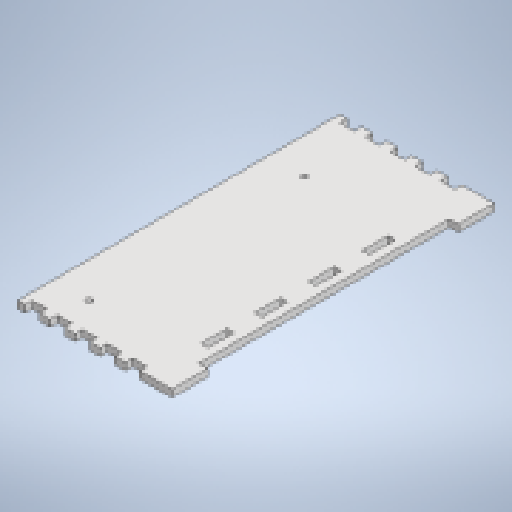
# Autodesk Inventor part: side
Saved by Autodesk Inventor 2025.3 (Build 293356000, 356)
## iProperties
Created: 2025-12-08
Part Number: side
Material: Generic
Document SubType Name: Modeling
Designer: hazem
Density: 1 g/cm^3
Appearance: Default
Author: hazem
Autodesk Inventor part; units mm, degrees
ref_plane "YZ Plane" through (0, 0, 0) normal (1, 0, 0) x (0, 1, 0)
ref_plane "XZ Plane" through (0, 0, 0) normal (0, 1, 0) x (-1, 0, 0)
ref_plane "XY Plane" through (0, 0, 0) normal (0, 0, 1) x (1, 0, 0)
sketch "Sketch1" plane through (0, 0, 0) normal (0, 1, 0) x (-1, 0, 0)
  line L0 (-9.6671, 163.8128) -> (70.4329, 163.8128)
  line L1 (70.4329, 163.8128) -> (70.4329, -16.1872)
  line L2 (70.4329, -16.1872) -> (-9.6671, -16.1872)
  line L3 (-9.6671, -16.1872) -> (-9.6671, 163.8128)
  point P0 (0, 0)
  constraints: 8 end point, 2 parallel, 1 horizontal, 1 perpendicular
extrude "Extrusion1" add sketch "Sketch1" along normal blind 4
sketch "Sketch2" plane through (0, 4, 0) normal (0, 1, 0) x (1, 0, 0)
  line L0 (-66.4329, -159.8128) -> (-66.4329, -148.8128)
  line L1 (-70.4329, -159.8128) -> (-70.4329, -148.8128)
  line L2 (-66.4329, -159.8128) -> (-66.4329, -148.8128) projected
  line L3 (-70.4329, -159.8128) -> (-70.4329, -148.8128) projected
  line L4 (-70.4329, -159.8128) -> (-70.4329, -148.8128) projected
  line L5 (-70.4329, -163.8128) -> (9.6671, -163.8128) projected
  line L6 (-30.3829, -163.8128) -> (-30.3829, 16.1872) construction
  line L7 (9.6671, 16.1872) -> (-70.4329, 16.1872) projected
  line L8 (-70.4329, 0.9372) -> (-66.4329, 0.9372)
  line L9 (-66.4329, -13.5628) -> (-70.4329, -13.5628)
  line L10 (-66.4329, -43.5628) -> (-70.4329, -43.5628)
  line L11 (-70.4329, -29.0628) -> (-66.4329, -29.0628)
  line L12 (-66.4329, -73.5628) -> (-70.4329, -73.5628)
  line L13 (-70.4329, -59.0628) -> (-66.4329, -59.0628)
  line L14 (-66.4329, -103.5628) -> (-70.4329, -103.5628)
  line L15 (-70.4329, -89.0628) -> (-66.4329, -89.0628)
  line L16 (-66.4329, -133.5628) -> (-70.4329, -133.5628)
  line L17 (-70.4329, -119.0628) -> (-66.4329, -119.0628)
  line L18 (5.6671, -159.8128) -> (5.6671, -148.8128)
  line L19 (9.6671, -159.8128) -> (9.6671, -148.8128)
  line L20 (5.6671, -133.8128) -> (5.6671, -118.8128)
  line L21 (9.6671, -133.8128) -> (9.6671, -118.8128)
  line L22 (5.6671, -103.8128) -> (5.6671, -88.8128)
  line L23 (9.6671, -103.8128) -> (9.6671, -88.8128)
  line L24 (5.6671, -73.8128) -> (5.6671, -58.8128)
  line L25 (9.6671, -73.8128) -> (9.6671, -58.8128)
  line L26 (5.6671, -43.8128) -> (5.6671, -28.8128)
  line L27 (9.6671, -43.8128) -> (9.6671, -28.8128)
  line L28 (5.6671, -13.8128) -> (5.6671, 1.1872)
  line L29 (9.6671, -13.8128) -> (9.6671, 1.1872)
  line L30 (9.6671, -149.0628) -> (5.6671, -149.0628)
  line L31 (5.6671, -159.5628) -> (9.6671, -159.5628)
  line L32 (9.6671, 0.9372) -> (5.6671, 0.9372)
  line L33 (5.6671, -13.5628) -> (9.6671, -13.5628)
  line L34 (5.6671, -43.5628) -> (9.6671, -43.5628)
  line L35 (9.6671, -29.0628) -> (5.6671, -29.0628)
  line L36 (5.6671, -73.5628) -> (9.6671, -73.5628)
  line L37 (9.6671, -59.0628) -> (5.6671, -59.0628)
  line L38 (5.6671, -103.5628) -> (9.6671, -103.5628)
  line L39 (9.6671, -89.0628) -> (5.6671, -89.0628)
  line L40 (5.6671, -133.5628) -> (9.6671, -133.5628)
  line L41 (9.6671, -119.0628) -> (5.6671, -119.0628)
  line L42 (-66.4329, -148.8128) -> (-70.4329, -148.8128)
  line L43 (-66.4329, -159.8128) -> (-70.4329, -159.8128)
  line L44 (-66.4329, -148.8128) -> (-70.4329, -148.8128)
  line L45 (-66.4329, -159.8128) -> (-70.4329, -159.8128) projected
  line L46 (-66.4329, -163.8128) -> (-66.4329, -89.0628)
  line L47 (-66.4329, -103.5628) -> (-66.4329, -73.5628)
  line L48 (-66.4329, -89.0628) -> (-66.4329, -43.5628)
  line L49 (-66.4329, -43.5628) -> (-66.4329, -13.5628)
  line L50 (-66.4329, -13.5628) -> (-66.4329, 16.1872)
  line L51 (-70.4329, 16.1872) -> (-70.4329, -163.8128) projected
  line L52 (9.6671, -163.8128) -> (9.6671, 16.1872) projected
  line L53 (1.6671, 16.1872) -> (1.6671, 12.1872)
  line L54 (1.6671, 12.1872) -> (-6.3329, 12.1872)
  line L55 (-6.3329, 12.1872) -> (-6.3329, 16.1872)
  line L56 (-12.3329, 16.1872) -> (-12.3329, 12.1872)
  line L57 (-12.3329, 12.1872) -> (-20.3329, 12.1872)
  line L58 (-20.3329, 12.1872) -> (-20.3329, 16.1872)
  line L59 (-26.3329, 16.1872) -> (-26.3329, 12.1872)
  line L60 (-26.3329, 12.1872) -> (-34.3329, 12.1872)
  line L61 (-34.3329, 12.1872) -> (-34.3329, 16.1872)
  line L62 (-40.3329, 16.1872) -> (-40.3329, 12.1872)
  line L63 (-40.3329, 12.1872) -> (-48.3329, 12.1872)
  line L64 (-48.3329, 12.1872) -> (-48.3329, 16.1872)
  line L65 (-54.3329, 16.1872) -> (-54.3329, 12.1872)
  line L66 (-54.3329, 12.1872) -> (-62.3329, 12.1872)
  line L67 (-62.3329, 12.1872) -> (-62.3329, 16.1872)
  line L68 (-12.3329, -73.8128) -> (-48.4329, -73.8128) construction
  line L69 (1.6671, -163.8128) -> (1.6671, -159.8128)
  line L70 (1.6671, -159.8128) -> (-6.3329, -159.8128)
  line L71 (-6.3329, -159.8128) -> (-6.3329, -163.8128)
  line L72 (-12.3329, -163.8128) -> (-12.3329, -159.8128)
  line L73 (-12.3329, -159.8128) -> (-20.3329, -159.8128)
  line L74 (-20.3329, -159.8128) -> (-20.3329, -163.8128)
  line L75 (-26.3329, -163.8128) -> (-26.3329, -159.8128)
  line L76 (-26.3329, -159.8128) -> (-34.3329, -159.8128)
  line L77 (-34.3329, -159.8128) -> (-34.3329, -163.8128)
  line L78 (-40.3329, -163.8128) -> (-40.3329, -159.8128)
  line L79 (-40.3329, -159.8128) -> (-48.3329, -159.8128)
  line L80 (-48.3329, -159.8128) -> (-48.3329, -163.8128)
  line L81 (-54.3329, -163.8128) -> (-54.3329, -159.8128)
  line L82 (-54.3329, -159.8128) -> (-62.3329, -159.8128)
  line L83 (-62.3329, -159.8128) -> (-62.3329, -163.8128)
  circle A0 centre (-46.4329, -23.8128) radius 1.75
  circle A1 centre (-46.4329, -143.8128) radius 1.75
  point P0 (0, 0)
  point P1 (-66.4329, -43.5628)
  point P2 (-30.3829, -73.8128)
  dimension "d6" = 30
  dimension "d13" = 4
  dimension "d14" = 8
  dimension "d15" = 4
  dimension "d16" = 8
  dimension "d19" = 14
  dimension "d24" = 180
  dimension "d30" = 3.5
  dimension "d32" = 40
  dimension "d34" = 20
  constraints: 152 end point, 44 symmetric about line, 21 point on line, 4 collinear, 4 midpoint, 3 vertical, 2 centre point, 2 horizontal, 1 equal radius, 1 parallel, 1 perpendicular, 1 vertical alignment, 54 other
  measures "d6" distance of L10.start L9.start
  measures "d13" distance of L53.start L53.end
  measures "d14" distance of L53.end L54.end
  measures "d15" distance of L54.end L55.end
  measures "d19" distance of L53.start L56.start
  measures "d24" distance between parallel lines of L5 L7
  measures "d30" diameter of A0
  measures "d32" distance from line of A0.centre L7
  measures "d34" distance from line of L5 A1.centre
extrude "Extrusion2" cut sketch "Sketch2" against normal up to surface (4 mm away) contours L43 L1 L42 L0 | L46 L5 L51 L43 | L42 L51 L16 L46 | L16 L51 L17 L46 | L83 L82 L81 L5 | L17 L51 L14 L46 | L14 L51 L15 L46 | L80 L79 L78 L5 | L15 L51 L12 L47 | L12 L51 L13 L48 | L77 L76 L75 L5 | L13 L51 L10 L48 | L10 L51 L11 L49 | L74 L73 L72 L5 | L11 L51 L9 L49 | L9 L51 L8 L50 | L71 L70 L69 L5 | L8 L51 L7 L50 | L7 L65 L66 L67 | L31 L18 L30 L19 | L7 L62 L63 L64 | L7 L59 L60 L61 | L40 L20 L41 L21 | L7 L56 L57 L58 | L7 L53 L54 L55 | L38 L22 L39 L23 | L29 L33 L28 L32 | L36 L24 L37 L25 | L27 L34 L26 L35 | A0 | A1
sketch "Sketch4" plane through (0, 4, 0) normal (0, 1, 0) x (1, 0, 0)
  line L0 (9.6671, -159.5628) -> (5.6671, -159.5628) projected
  line L1 (9.6671, -149.0628) -> (9.6671, -133.5628) projected
  line L2 (5.6671, -159.5628) -> (9.6671, -159.5628)
  line L3 (9.6671, -159.5628) -> (9.6671, -149.0628)
  line L4 (9.6671, -149.0628) -> (5.6671, -149.0628)
  line L5 (5.6671, -149.0628) -> (5.6671, -159.5628)
  line L6 (5.6671, -13.5628) -> (5.6671, 0.9372) projected
  line L7 (9.6671, -13.5628) -> (5.6671, -13.5628)
  line L8 (5.6671, -13.5628) -> (5.6671, 0.9372)
  line L9 (5.6671, 0.9372) -> (9.6671, 0.9372)
  line L10 (9.6671, 0.9372) -> (9.6671, -133.5628)
  line L11 (9.6671, -13.5628) -> (5.6671, -13.5628) projected
  line L12 (1.6671, -163.8128) -> (9.6671, -163.8128) projected
  line L13 (9.6671, -163.8128) -> (19.6671, -163.8128)
  line L14 (19.6671, -163.8128) -> (19.6671, -143.8128)
  line L15 (19.6671, -143.8128) -> (9.6671, -143.8128)
  line L16 (9.6671, -143.8128) -> (9.6671, -163.8128)
  line L17 (9.6671, 16.1872) -> (1.6671, 16.1872) projected
  line L18 (9.6671, 16.1872) -> (19.6671, 16.1872)
  line L19 (19.6671, 16.1872) -> (19.6671, -3.8128)
  line L20 (19.6671, -3.8128) -> (9.6671, -3.8128)
  line L21 (9.6671, -3.8128) -> (9.6671, 16.1872)
  line L22 (14.6671, -143.8128) -> (14.6671, -3.8128)
  line L23 (-40.3329, -159.8128) -> (-40.3329, -163.8128) projected
  line L24 (-40.3329, -163.8128) -> (-34.3329, -163.8128) projected
  line L25 (-34.3329, -163.8128) -> (-34.3329, -159.8128) projected
  line L26 (-34.3329, -159.8128) -> (-26.3329, -159.8128) projected
  line L27 (-26.3329, -159.8128) -> (-26.3329, -163.8128) projected
  line L28 (-26.3329, -163.8128) -> (-20.3329, -163.8128) projected
  line L29 (-20.3329, -163.8128) -> (-20.3329, -159.8128) projected
  line L30 (-20.3329, -159.8128) -> (-12.3329, -159.8128) projected
  line L31 (-12.3329, -159.8128) -> (-12.3329, -163.8128) projected
  line L32 (-12.3329, -163.8128) -> (-6.3329, -163.8128) projected
  line L33 (-6.3329, -163.8128) -> (-6.3329, -159.8128) projected
  line L34 (-6.3329, -159.8128) -> (1.6671, -159.8128) projected
  line L35 (1.6671, -159.8128) -> (1.6671, -163.8128) projected
  line L36 (1.6671, -163.8128) -> (9.6671, -163.8128) projected
  line L37 (9.6671, -163.8128) -> (9.6671, -159.5628) projected
  line L38 (9.6671, -159.5628) -> (5.6671, -159.5628) projected
  line L39 (5.6671, -159.5628) -> (5.6671, -149.0628) projected
  line L40 (5.6671, -149.0628) -> (9.6671, -149.0628) projected
  line L41 (9.6671, -149.0628) -> (9.6671, -133.5628) projected
  line L42 (9.6671, -133.5628) -> (5.6671, -133.5628) projected
  line L43 (5.6671, -133.5628) -> (5.6671, -119.0628) projected
  line L44 (5.6671, -119.0628) -> (9.6671, -119.0628) projected
  line L45 (9.6671, -119.0628) -> (9.6671, -103.5628) projected
  line L46 (9.6671, -103.5628) -> (5.6671, -103.5628) projected
  line L47 (5.6671, -103.5628) -> (5.6671, -89.0628) projected
  line L48 (5.6671, -89.0628) -> (9.6671, -89.0628) projected
  line L49 (9.6671, -89.0628) -> (9.6671, -73.5628) projected
  line L50 (9.6671, -73.5628) -> (5.6671, -73.5628) projected
  line L51 (5.6671, -73.5628) -> (5.6671, -59.0628) projected
  line L52 (5.6671, -59.0628) -> (9.6671, -59.0628) projected
  line L53 (9.6671, -59.0628) -> (9.6671, -43.5628) projected
  line L54 (9.6671, -43.5628) -> (5.6671, -43.5628) projected
  line L55 (5.6671, -43.5628) -> (5.6671, -29.0628) projected
  line L56 (5.6671, -29.0628) -> (9.6671, -29.0628) projected
  line L57 (9.6671, -29.0628) -> (9.6671, -13.5628) projected
  line L58 (9.6671, -13.5628) -> (5.6671, -13.5628) projected
  line L59 (5.6671, -13.5628) -> (5.6671, 0.9372) projected
  line L60 (5.6671, 0.9372) -> (9.6671, 0.9372) projected
  line L61 (9.6671, 0.9372) -> (9.6671, 16.1872) projected
  line L62 (9.6671, 16.1872) -> (1.6671, 16.1872) projected
  line L63 (1.6671, 16.1872) -> (1.6671, 12.1872) projected
  line L64 (1.6671, 12.1872) -> (-6.3329, 12.1872) projected
  line L65 (-6.3329, 12.1872) -> (-6.3329, 16.1872) projected
  line L66 (-6.3329, 16.1872) -> (-12.3329, 16.1872) projected
  line L67 (-12.3329, 16.1872) -> (-12.3329, 12.1872) projected
  line L68 (-12.3329, 12.1872) -> (-20.3329, 12.1872) projected
  line L69 (-20.3329, 12.1872) -> (-20.3329, 16.1872) projected
  line L70 (-20.3329, 16.1872) -> (-26.3329, 16.1872) projected
  line L71 (-26.3329, 16.1872) -> (-26.3329, 12.1872) projected
  line L72 (-26.3329, 12.1872) -> (-34.3329, 12.1872) projected
  line L73 (-34.3329, 12.1872) -> (-34.3329, 16.1872) projected
  line L74 (-34.3329, 16.1872) -> (-40.3329, 16.1872) projected
  line L75 (-40.3329, 16.1872) -> (-40.3329, 12.1872) projected
  line L76 (-40.3329, 12.1872) -> (-48.3329, 12.1872) projected
  line L77 (-48.3329, 12.1872) -> (-48.3329, 16.1872) projected
  line L78 (-48.3329, 16.1872) -> (-54.3329, 16.1872) projected
  line L79 (-54.3329, 16.1872) -> (-54.3329, 12.1872) projected
  line L80 (-54.3329, 12.1872) -> (-62.3329, 12.1872) projected
  line L81 (-62.3329, 12.1872) -> (-62.3329, 16.1872) projected
  line L82 (-62.3329, 16.1872) -> (-66.4329, 16.1872) projected
  line L83 (-66.4329, -163.8128) -> (-62.3329, -163.8128) projected
  line L84 (-62.3329, -163.8128) -> (-62.3329, -159.8128) projected
  line L85 (-62.3329, -159.8128) -> (-54.3329, -159.8128) projected
  line L86 (-54.3329, -159.8128) -> (-54.3329, -163.8128) projected
  line L87 (-54.3329, -163.8128) -> (-48.3329, -163.8128) projected
  line L88 (-48.3329, -163.8128) -> (-48.3329, -159.8128) projected
  line L89 (-48.3329, -159.8128) -> (-40.3329, -159.8128) projected
  line L90 (-66.4329, 16.1872) -> (-66.4329, -163.8128) projected
  point P0 (0, 0)
  dimension "d25" = 10
  dimension "d26" = 20
  dimension "d29" = 5
  constraints: 34 end point, 8 parallel, 5 perpendicular, 4 horizontal, 3 point on line, 2 equal length, 2 midpoint, 1 collinear
  measures "d25" distance of L15.end L14.end
  measures "d26" distance of L14.end L13.end
  measures "d29" distance between parallel lines of L1 L22
extrude "Extrusion3" add sketch "Sketch4" against normal up to surface (4 mm away) contours L0 L5 L4 L3 | L3 L1 L15 L14 L13 L16 | L1 L10 L20 L22 L15 | L20 L10 L21 L18 L19 | L10 L7 L6 L9
body "Solid1"
